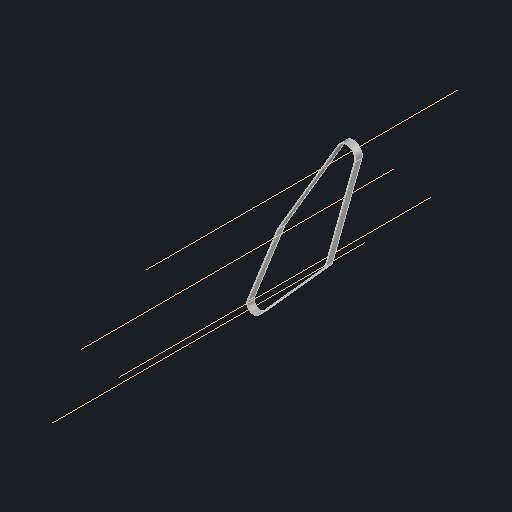
# Autodesk Inventor part: Зубчатый ремень
Saved by Autodesk Inventor 2024 (Build 280153000, 153)
## iProperties
Created: 2023-09-26
Part Number: Зубчатый ремень
Material: Rubber
Document SubType Name: Modeling
Designer: user
Density: 1 g/cm^3
Appearance: Rubber - Black - Version 1.1
CustomPartVersion: 1
Author: user
Autodesk Inventor part; units mm, degrees
sketch "Эскизная траектория" plane through (0, 0, 0) normal (0, 0, 1) x (1, 0, 0)
  arc A0 (-12.322302, 6.766147) -> (-2.030215, 0.411254) centre (-6.605836, 4.51253) ccw
  arc A1 (16.421153, 79.531094) -> (16.125565, 78.926271) centre (20.090569, 77.363138) ccw
  arc A2 (87.840901, 169.167002) -> (73.09156, 175.449677) centre (80.052491, 171.337035) ccw
  arc A3 (59.329742, 68.867976) -> (60.480315, 70.9678) centre (55.41139, 72.38012) ccw
  line L0 (59.329742, 68.867976) -> (-2.030215, 0.411254)
  line L1 (-12.322302, 6.766147) -> (16.125565, 78.926271)
  line L2 (16.421153, 79.531094) -> (73.09156, 175.449677)
  line L3 (87.840901, 169.167002) -> (60.480315, 70.9678)
  constraints: 8 end point, 8 point on circle, 4 centre point
ref_plane "Плоскость сечения" through (-2.030215, 0.411254, 0) normal (0.6674543, 0.7446507, 0) x (0, 0, 1)
ref_plane "РабПлоскость2" through (-6.605836, 4.51253, 0) normal (-1, 0, 0) x (0, 0, 1)
ref_plane "РабПлоскость3" through (80.052491, 171.337035, 0) normal (-0.53125, -0.8472151, 0) x (0, 0, 1)
sketch "Сечение" plane through (-2.030215, 0.411254, 0) normal (0.6674543, 0.7446507, 0) x (0, 0, 1)
  line L0 (-3.175, 0.381) -> (3.175, 0.381)
  line L1 (3.175, 0.381) -> (3.175, -0.254)
  line L2 (3.175, -0.254) -> (-3.175, -0.254)
  line L3 (-3.175, -0.254) -> (-3.175, 0.381)
  line L4 (-3.175, 0) -> (3.175, 0) construction
  point P0 (0, 0)
  point P1 (0, 0)
  dimension "d0" = 6.35
  dimension "d4" = 0.254
  dimension "d5" = 0.381
  constraints: 10 end point, 2 parallel, 2 point on line, 1 coincident, 1 horizontal, 1 midpoint, 1 perpendicular, 1 other
  measures "d0" distance between parallel lines of L1 L3
  measures "d4" distance between parallel lines of L2 L4
  measures "d5" distance between parallel lines of L4 L0
sweep "Ремень" add profiles "Сечение" path "Эскизная траектория"
equation "\"d0\" = da_B"
equation "\"d4\" = da_a"
equation "\"d5\" = da_a2"
equation "\"da_B\" = 6.35"
equation "\"da_pb\" = 2.032"
equation "\"da_L\" = 426.33783"
equation "\"da_a\" = 0.254"
equation "\"da_S\" = 1.143"
equation "\"da_Beta\" = 20deg"
equation "\"da_Ht\" = 0.508"
equation "\"da_H\" = 1.143"
equation "\"da_a2\" = 0.381"
body "Solid1"
